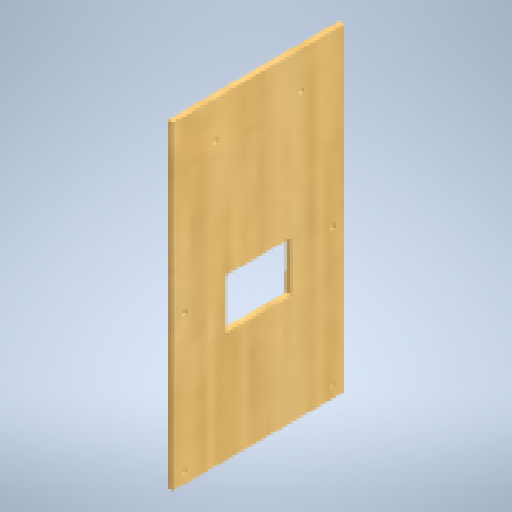
# Autodesk Inventor part: Panel3
Saved by Autodesk Inventor 2023 (Build 270158000, 158)
## iProperties
Created: 2022-12-03
Part Number: Panel3
Material: Genérico
Document SubType Name: Modeling
Designer: sergi
Density: 1 g/cm^3
Appearance: Valor por defecto
Author: sergi
Autodesk Inventor part; units mm, degrees
ref_plane "YZ Plane" through (0, 0, 0) normal (1, 0, 0) x (0, 1, 0)
ref_plane "XZ Plane" through (0, 0, 0) normal (0, 1, 0) x (-1, 0, 0)
ref_plane "XY Plane" through (0, 0, 0) normal (0, 0, 1) x (1, 0, 0)
sketch "Boceto1" plane through (0, 0, 0) normal (0, 1, 0) x (-1, 0, 0)
  line L0 (-1.5, -48.5) -> (1.5, -48.5)
  line L1 (1.5, -48.5) -> (1.5, 48.5)
  line L2 (1.5, 48.5) -> (-1.5, 48.5)
  line L3 (-1.5, 48.5) -> (-1.5, -48.5)
  line L4 (-1.5, -48.5) -> (1.5, 48.5) construction
  line L5 (1.5, -48.5) -> (-1.5, 48.5) construction
  point P0 (0, 0)
  dimension "d0" = 3
  dimension "d1" = 97
  constraints: 12 end point, 2 midpoint, 2 parallel, 1 horizontal, 1 perpendicular
  measures "d0" distance of L2.end L1.end
  measures "d1" distance of L1.end L0.end
extrude "Extrusión1" add sketch "Boceto1" along normal blind 180
sketch "Boceto2" plane through (-1.5, 0, -48.5) normal (-1, 0, 0) x (0, 0, 1)
  line L0 (97, 90.5) -> (0, 90.5)
  circle A0 centre (23.1283, 84.5) radius 1.25 projected
  circle A1 centre (73.8717, 84.5) radius 1.25 projected
  line L1 (30.1317, 63.5948) -> (30.1317, 90.5)
  line L2 (66.8717, 90.5) -> (66.8717, 63.5948)
  line L3 (66.8717, 63.5948) -> (30.1317, 63.5948) projected
  line L4 (30.1317, 63.5948) -> (30.1317, 90.5) projected
  line L5 (66.8717, 90.5) -> (66.8717, 63.5948) projected
  point P0 (48.5, 0)
  constraints: 6 end point, 3 point on line
extrude "Extrusión2" cut sketch "Boceto2" against normal through all contours L2 L3 L1 L0
sketch "Boceto3" plane through (-1.5, 0, -48.5) normal (-1, 0, 0) x (0, 0, 1)
  circle A0 centre (6.5, 6.5) radius 1.25 projected
  circle A1 centre (90.5, 6.5) radius 1.25 projected
  circle A2 centre (90.5, 84) radius 1.5 projected
  circle A3 centre (6.5, 84) radius 1.5 projected
  point P0 (48.5, 0)
extrude "Extrusión3" cut sketch "Boceto3" against normal through all
sketch "Boceto4" plane through (-1.5, 0, -48.5) normal (-1, 0, 0) x (0, 0, 1)
  line L0 (80, 148.5) -> (17, 148.5) projected
  line L1 (0, 148.5) -> (97, 148.5) projected
  line L2 (6.3714, 170) -> (90.6286, 170) projected
  line L3 (48.5, 148.5) -> (48.5, 170)
  line L4 (48.5, 159.25) -> (24.25, 159.25)
  line L5 (24.25, 159.25) -> (72.75, 159.25)
  circle A0 centre (24.25, 159.25) radius 1.5
  circle A1 centre (72.75, 159.25) radius 1.5
  point P0 (48.5, 0)
  dimension "d8" = 24.25
  dimension "d9" = 48.5
  dimension "d10" = 3
  dimension "d11" = 3
  constraints: 6 end point, 3 midpoint, 2 centre point, 2 coincident, 1 horizontal, 1 point on line
  measures "d8" distance of L4.start L4.end
  measures "d9" distance of L4.end L5.end
  measures "d10" diameter of A0
  measures "d11" diameter of A1
hole "Agujero1" at (-1.5, 159.25, -24.25) at (-1.5, 159.25, 24.25) direction (1, 0, 0) diameter 3 end through all
